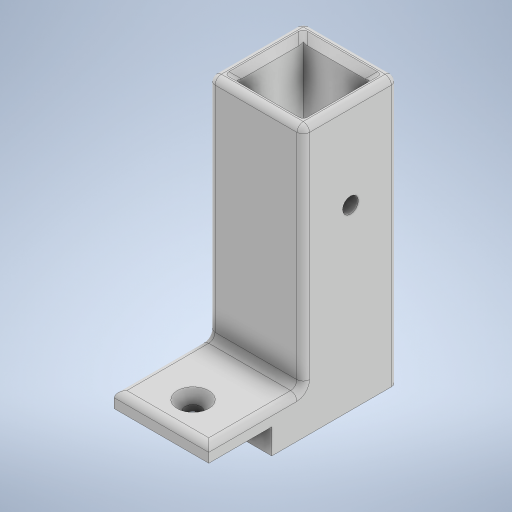
# Autodesk Inventor part: flexibler_standfuß_v0.8
Saved by Autodesk Inventor 2024 (Build 280153000, 153)
## iProperties
Created: 2023-12-27
Part Number: flexibler_standfuß_v0.8
Material: Generic
Document SubType Name: Modeling
Designer: Julian
Density: 1 g/cm^3
Appearance: Default
Author: Julian
Autodesk Inventor part; units mm, degrees
ref_plane "YZ Plane" through (0, 0, 0) normal (1, 0, 0) x (0, 1, 0)
ref_plane "XZ Plane" through (0, 0, 0) normal (0, 1, 0) x (-1, 0, 0)
ref_plane "XY Plane" through (0, 0, 0) normal (0, 0, 1) x (1, 0, 0)
sketch "Sketch1" plane through (0, 0, 0) normal (1, 0, 0) x (0, 1, 0)
  line L0 (0, 0) -> (0, -30)
  line L1 (13, 0) -> (30, 0) construction
  line L2 (0, -30) -> (85, -30)
  line L3 (13, 0) -> (85, 0)
  line L4 (85, 0) -> (85, -30)
  line L5 (0, 0) -> (0, 10)
  line L6 (13, 0) -> (14, 0) construction
  line L7 (0, 10) -> (8, 10)
  line L8 (8, 10) -> (8, 30)
  line L9 (8, 30) -> (13, 30)
  line L10 (13, 30) -> (13, 0)
  point P0 (59, -15)
  dimension "d0" = 30
  dimension "d2" = 85
  dimension "d4" = 10
  dimension "d6" = 8
  dimension "d7" = 20
  dimension "d8" = 5
  dimension "d47" = 30
  constraints: 22 end point, 4 horizontal, 4 vertical, 1 perpendicular, 1 point on line
  measures "d0" distance of L0.start L0.end
  measures "d2" distance of L0.end L2.end
  measures "d4" distance of L0.start L5.end
  measures "d6" distance of L5.end L7.end
  measures "d7" distance of L7.end L8.end
  measures "d8" distance of L8.end L9.end
  measures "d47" distance between parallel lines of L2 L3
extrude "Extrusion1" add sketch "Sketch1" along normal blind 30
sketch "Sketch2" plane through (0, 85, 0) normal (0, 1, 0) x (1, 0, 0)
  line L0 (4.5, 4.5) -> (4.5, 25.5)
  line L1 (4.5, 4.5) -> (25.5, 4.5) construction
  line L2 (4.5, 25.5) -> (25.5, 25.5)
  line L3 (25.5, 25.5) -> (25.5, 4.5)
  line L4 (25.5, 4.5) -> (4.5, 4.5)
  line L5 (30, 30) -> (30, 0) projected
  point P0 (0, 0)
  dimension "d13" = 21
  dimension "d14" = 90
  dimension "d15" = 21
  dimension "d16" = 90
  dimension "d17" = 21
  dimension "d18" = 90
  dimension "d19" = 21
  dimension "d46" = 4.5
  dimension "d48" = 90
  dimension "d49" = 4.5
  constraints: 10 end point, 3 perpendicular, 1 horizontal, 1 vertical
  measures "d13" distance of L0.start L0.end
  measures "d14" angle of L1 L0
  measures "d15" distance of L0.end L2.end
  measures "d16" angle of L0 L2
  measures "d17" distance of L2.end L3.end
  measures "d18" angle of L2 L3
  measures "d19" distance of L3.end L0.start
  measures "d46" distance from line of L1 point (0, 0)
  measures "d48" angle of L1 L3
  measures "d49" distance between parallel lines of L5 L3
extrude "Extrusion2" cut sketch "Sketch2" against normal blind 80
fillet "Fillet1" radius 2 12 edges at (30, 85, -15) (15, 85, 0) (15, 85, -30) (0, 85, -15) (30, 49, 0) (30, 42.5, -30) (0, 49, 0) (0, 42.5, -30) (0, 13, 15) (15, 13, 30) (30, 13, 15) (15, 13, 0)
sketch "Sketch4" plane through (2, 13, 2) normal (0, 1, 0) x (1, 0, 0)
  line L0 (-2, -28) -> (28, -28) projected
  point P0 (-2, 2)
  point P1 (13, -18)
  point P2 (13, -28)
  dimension "d37" = 10
  constraints: 1 midpoint
  measures "d37" distance of point (13, -28) point (13, -18)
hole "Hole1" at (15, 13, 20) direction (0, -1, 0) diameter 5 end through all countersink diameter 10 countersink angle 77.33
sketch "Sketch6" plane through (30, 0, 0) normal (1, 0, 0) x (0, 0, -1)
  line L0 (-10, 0) -> (28, 0) projected
  point P0 (0, 0)
  point P1 (15, 56.5)
  dimension "d45" = 56.5
  measures "d45" distance from line of L0 point (15, 56.5)
hole "Hole2" at (30, 56.5, -15) direction (-1, 0, 0) diameter 5 end through all
chamfer "Chamfer2" distance 2 angle 45 4 edges at (4.5, 85, -15) (15, 85, -25.5) (25.5, 85, -15) (15, 85, -4.5)
fillet "Fillet3" radius 2 4 edges at (3.5, 84, -26.5) (26.5, 84, -26.5) (26.5, 84, -3.5) (3.5, 84, -3.5)
body "Solid1"
